Autodesk Fusion 360 part; units mm, degrees
(part 2 of 2)
extrude "Extrude179" add sketch "Sketch179" along normal blind 62 from surface at 3 bodies 3
sketch "Sketch180" plane through (0, 0, 0) normal (0, 0, 1) x (1, 0, 0)
  line L0 (-121.5, 16) -> (-128.5, 16)
  line L1 (-128.5, 16) -> (-128.5, 3)
  line L2 (-128.5, 3) -> (-121.5, 3)
  line L3 (-121.5, 3) -> (-121.5, 16)
extrude "Extrude180" add sketch "Sketch180" along normal blind 8 from surface at 57 bodies 3
sketch "Sketch181" plane through (0, 0, 0) normal (0, 0, 1) x (1, 0, 0)
  circle A0 centre (-125, 12) radius 1.3
extrude "Extrude181" cut sketch "Sketch181" along normal blind 8 from surface at 57 bodies 3
sketch "Sketch182" plane through (0, 0, 0) normal (0, 0, 1) x (1, 0, 0)
  line L0 (128.5, 16) -> (121.5, 16)
  line L1 (121.5, 16) -> (121.5, 3)
  line L2 (121.5, 3) -> (128.5, 3)
  line L3 (128.5, 3) -> (128.5, 16)
extrude "Extrude182" add sketch "Sketch182" along normal blind 8 from surface at 57 bodies 3
sketch "Sketch183" plane through (0, 0, 0) normal (0, 0, 1) x (1, 0, 0)
  circle A0 centre (125, 12) radius 1.3
extrude "Extrude183" cut sketch "Sketch183" along normal blind 8 from surface at 57 bodies 3
sketch "Sketch184" plane through (0, 0, 0) normal (0, 0, 1) x (1, 0, 0)
  line L0 (140, 83) -> (-140, 83)
  line L1 (-140, 83) -> (-140, 80)
  line L2 (-140, 80) -> (140, 80)
  line L3 (140, 80) -> (140, 83)
extrude "Extrude184" add sketch "Sketch184" along normal blind 3 bodies 3
sketch "Sketch185" plane through (0, 0, 0) normal (0, 0, 1) x (1, 0, 0)
  line L0 (125, 82.3) -> (-125, 82.3)
  line L1 (-125, 82.3) -> (-125, 80.7)
  line L2 (-125, 80.7) -> (125, 80.7)
  line L3 (125, 80.7) -> (125, 82.3)
extrude "Extrude185" cut sketch "Sketch185" along normal blind 2 from surface at 2 bodies 3
move_body "Move2" bodies 3 to x (-1, 0, 0) y (0, 0, 1) z (0, 1, 0) at (0, 137, 0)
sketch "Sketch186" plane through (0, 0, 0) normal (0, 0, 1) x (1, 0, 0)
  line L0 (140, 40) -> (-140, 40)
  line L1 (-140, 40) -> (-140, -40)
  line L2 (-140, -40) -> (140, -40)
  line L3 (140, -40) -> (140, 40)
extrude "Extrude186" add sketch "Sketch186" along normal blind 2.5 separate body makes body 4
sketch "Sketch187" plane through (0, 0, 0) normal (0, 0, 1) x (1, 0, 0)
  line L0 (94, -33) -> (87, -33)
  line L1 (87, -33) -> (87, -42)
  line L2 (87, -42) -> (94, -42)
  line L3 (94, -42) -> (94, -33)
extrude "Extrude187" cut sketch "Sketch187" along normal blind 2.95 from surface at -1 bodies 4
sketch "Sketch188" plane through (0, 0, 0) normal (0, 0, 1) x (1, 0, 0)
  circle A0 centre (90.5, -33) radius 3.5
extrude "Extrude188" cut sketch "Sketch188" along normal blind 2.95 from surface at -1 bodies 4
sketch "Sketch189" plane through (0, 0, 0) normal (0, 0, 1) x (1, 0, 0)
  line L0 (80, -33) -> (73, -33)
  line L1 (73, -33) -> (73, -42)
  line L2 (73, -42) -> (80, -42)
  line L3 (80, -42) -> (80, -33)
extrude "Extrude189" cut sketch "Sketch189" along normal blind 2.95 from surface at -1 bodies 4
sketch "Sketch190" plane through (0, 0, 0) normal (0, 0, 1) x (1, 0, 0)
  circle A0 centre (76.5, -33) radius 3.5
extrude "Extrude190" cut sketch "Sketch190" along normal blind 2.95 from surface at -1 bodies 4
sketch "Sketch191" plane through (0, 0, 0) normal (0, 0, 1) x (1, 0, 0)
  line L0 (66, -33) -> (59, -33)
  line L1 (59, -33) -> (59, -42)
  line L2 (59, -42) -> (66, -42)
  line L3 (66, -42) -> (66, -33)
extrude "Extrude191" cut sketch "Sketch191" along normal blind 2.95 from surface at -1 bodies 4
sketch "Sketch192" plane through (0, 0, 0) normal (0, 0, 1) x (1, 0, 0)
  circle A0 centre (62.5, -33) radius 3.5
extrude "Extrude192" cut sketch "Sketch192" along normal blind 2.95 from surface at -1 bodies 4
sketch "Sketch193" plane through (0, 0, 0) normal (0, 0, 1) x (1, 0, 0)
  line L0 (52, -33) -> (45, -33)
  line L1 (45, -33) -> (45, -42)
  line L2 (45, -42) -> (52, -42)
  line L3 (52, -42) -> (52, -33)
extrude "Extrude193" cut sketch "Sketch193" along normal blind 2.95 from surface at -1 bodies 4
sketch "Sketch194" plane through (0, 0, 0) normal (0, 0, 1) x (1, 0, 0)
  circle A0 centre (48.5, -33) radius 3.5
extrude "Extrude194" cut sketch "Sketch194" along normal blind 2.95 from surface at -1 bodies 4
sketch "Sketch195" plane through (0, 0, 0) normal (0, 0, 1) x (1, 0, 0)
  line L0 (38, -33) -> (31, -33)
  line L1 (31, -33) -> (31, -42)
  line L2 (31, -42) -> (38, -42)
  line L3 (38, -42) -> (38, -33)
extrude "Extrude195" cut sketch "Sketch195" along normal blind 2.95 from surface at -1 bodies 4
sketch "Sketch196" plane through (0, 0, 0) normal (0, 0, 1) x (1, 0, 0)
  circle A0 centre (34.5, -33) radius 3.5
extrude "Extrude196" cut sketch "Sketch196" along normal blind 2.95 from surface at -1 bodies 4
sketch "Sketch197" plane through (0, 0, 0) normal (0, 0, 1) x (1, 0, 0)
  line L0 (-99.5, -33) -> (-106.5, -33)
  line L1 (-106.5, -33) -> (-106.5, -42)
  line L2 (-106.5, -42) -> (-99.5, -42)
  line L3 (-99.5, -42) -> (-99.5, -33)
extrude "Extrude197" cut sketch "Sketch197" along normal blind 2.95 from surface at -1 bodies 4
sketch "Sketch198" plane through (0, 0, 0) normal (0, 0, 1) x (1, 0, 0)
  circle A0 centre (-103, -33) radius 3.5
extrude "Extrude198" cut sketch "Sketch198" along normal blind 2.95 from surface at -1 bodies 4
sketch "Sketch199" plane through (0, 0, 0) normal (0, 0, 1) x (1, 0, 0)
  line L0 (-83.5, -33) -> (-90.5, -33)
  line L1 (-90.5, -33) -> (-90.5, -42)
  line L2 (-90.5, -42) -> (-83.5, -42)
  line L3 (-83.5, -42) -> (-83.5, -33)
extrude "Extrude199" cut sketch "Sketch199" along normal blind 2.95 from surface at -1 bodies 4
sketch "Sketch200" plane through (0, 0, 0) normal (0, 0, 1) x (1, 0, 0)
  circle A0 centre (-87, -33) radius 3.5
extrude "Extrude200" cut sketch "Sketch200" along normal blind 2.95 from surface at -1 bodies 4
sketch "Sketch201" plane through (0, 0, 0) normal (0, 0, 1) x (1, 0, 0)
  line L0 (-67.5, -33) -> (-74.5, -33)
  line L1 (-74.5, -33) -> (-74.5, -42)
  line L2 (-74.5, -42) -> (-67.5, -42)
  line L3 (-67.5, -42) -> (-67.5, -33)
extrude "Extrude201" cut sketch "Sketch201" along normal blind 2.95 from surface at -1 bodies 4
sketch "Sketch202" plane through (0, 0, 0) normal (0, 0, 1) x (1, 0, 0)
  circle A0 centre (-71, -33) radius 3.5
extrude "Extrude202" cut sketch "Sketch202" along normal blind 2.95 from surface at -1 bodies 4
sketch "Sketch203" plane through (0, 0, 0) normal (0, 0, 1) x (1, 0, 0)
  line L0 (-51.5, -33) -> (-58.5, -33)
  line L1 (-58.5, -33) -> (-58.5, -42)
  line L2 (-58.5, -42) -> (-51.5, -42)
  line L3 (-51.5, -42) -> (-51.5, -33)
extrude "Extrude203" cut sketch "Sketch203" along normal blind 2.95 from surface at -1 bodies 4
sketch "Sketch204" plane through (0, 0, 0) normal (0, 0, 1) x (1, 0, 0)
  circle A0 centre (-55, -33) radius 3.5
extrude "Extrude204" cut sketch "Sketch204" along normal blind 2.95 from surface at -1 bodies 4
sketch "Sketch205" plane through (0, 0, 0) normal (0, 0, 1) x (1, 0, 0)
  line L0 (-35.5, -33) -> (-42.5, -33)
  line L1 (-42.5, -33) -> (-42.5, -42)
  line L2 (-42.5, -42) -> (-35.5, -42)
  line L3 (-35.5, -42) -> (-35.5, -33)
extrude "Extrude205" cut sketch "Sketch205" along normal blind 2.95 from surface at -1 bodies 4
sketch "Sketch206" plane through (0, 0, 0) normal (0, 0, 1) x (1, 0, 0)
  circle A0 centre (-39, -33) radius 3.5
extrude "Extrude206" cut sketch "Sketch206" along normal blind 2.95 from surface at -1 bodies 4
sketch "Sketch207" plane through (0, 0, 0) normal (0, 0, 1) x (1, 0, 0)
  line L0 (-6.5, -33) -> (-13.5, -33)
  line L1 (-13.5, -33) -> (-13.5, -42)
  line L2 (-13.5, -42) -> (-6.5, -42)
  line L3 (-6.5, -42) -> (-6.5, -33)
extrude "Extrude207" cut sketch "Sketch207" along normal blind 2.95 from surface at -1 bodies 4
sketch "Sketch208" plane through (0, 0, 0) normal (0, 0, 1) x (1, 0, 0)
  circle A0 centre (-10, -33) radius 3.5
extrude "Extrude208" cut sketch "Sketch208" along normal blind 2.95 from surface at -1 bodies 4
sketch "Sketch209" plane through (0, 0, 0) normal (0, 0, 1) x (1, 0, 0)
  line L0 (140, 40) -> (-140, 40)
  line L1 (-140, 40) -> (-140, 37.5)
  line L2 (-140, 37.5) -> (140, 37.5)
  line L3 (140, 37.5) -> (140, 40)
extrude "Extrude209" add sketch "Sketch209" along normal blind 65 bodies 4
sketch "Sketch210" plane through (0, 0, 0) normal (0, 0, 1) x (1, 0, 0)
  line L0 (124.5, 39) -> (-124.5, 39)
  line L1 (-124.5, 39) -> (-124.5, 38)
  line L2 (-124.5, 38) -> (124.5, 38)
  line L3 (124.5, 38) -> (124.5, 39)
extrude "Extrude210" add sketch "Sketch210" along normal blind 0.7 from surface at 65 bodies 4
sketch "Sketch211" plane through (0, 0, 0) normal (0, 0, 1) x (1, 0, 0)
  line L0 (-137.5, 40) -> (-140, 40)
  line L1 (-140, 40) -> (-140, -40)
  line L2 (-140, -40) -> (-137.5, -40)
  line L3 (-137.5, -40) -> (-137.5, 40)
extrude "Extrude211" add sketch "Sketch211" along normal blind 65 bodies 4
sketch "Sketch212" plane through (0, 0, 0) normal (0, 0, 1) x (1, 0, 0)
  line L0 (140, 40) -> (137.5, 40)
  line L1 (137.5, 40) -> (137.5, -40)
  line L2 (137.5, -40) -> (140, -40)
  line L3 (140, -40) -> (140, 40)
extrude "Extrude212" add sketch "Sketch212" along normal blind 65 bodies 4
sketch "Sketch213" plane through (0, 0, 0) normal (0, 0, 1) x (1, 0, 0)
  line L0 (-129.1, -31.7) -> (-136.9, -31.7)
  line L1 (-136.9, -31.7) -> (-136.9, -34.7)
  line L2 (-136.9, -34.7) -> (-129.1, -34.7)
  line L3 (-129.1, -34.7) -> (-129.1, -31.7)
extrude "Extrude213" add sketch "Sketch213" along normal blind 60.5 from surface at 2.5 bodies 4
sketch "Sketch214" plane through (0, 0, 0) normal (0, 0, 1) x (1, 0, 0)
  line L0 (-135.3, -34.7) -> (-136.9, -34.7)
  line L1 (-136.9, -34.7) -> (-136.9, -40)
  line L2 (-136.9, -40) -> (-135.3, -40)
  line L3 (-135.3, -40) -> (-135.3, -34.7)
extrude "Extrude214" add sketch "Sketch214" along normal blind 60.5 from surface at 2.5 bodies 4
sketch "Sketch215" plane through (0, 0, 0) normal (0, 0, 1) x (1, 0, 0)
  line L0 (-129.1, -34.7) -> (-130.7, -34.7)
  line L1 (-130.7, -34.7) -> (-130.7, -40)
  line L2 (-130.7, -40) -> (-129.1, -40)
  line L3 (-129.1, -40) -> (-129.1, -34.7)
extrude "Extrude215" add sketch "Sketch215" along normal blind 60.5 from surface at 2.5 bodies 4
sketch "Sketch216" plane through (0, 0, 0) normal (0, 0, 1) x (1, 0, 0)
  line L0 (136.9, -31.7) -> (129.1, -31.7)
  line L1 (129.1, -31.7) -> (129.1, -34.7)
  line L2 (129.1, -34.7) -> (136.9, -34.7)
  line L3 (136.9, -34.7) -> (136.9, -31.7)
extrude "Extrude216" add sketch "Sketch216" along normal blind 60.5 from surface at 2.5 bodies 4
sketch "Sketch217" plane through (0, 0, 0) normal (0, 0, 1) x (1, 0, 0)
  line L0 (130.7, -34.7) -> (129.1, -34.7)
  line L1 (129.1, -34.7) -> (129.1, -40)
  line L2 (129.1, -40) -> (130.7, -40)
  line L3 (130.7, -40) -> (130.7, -34.7)
extrude "Extrude217" add sketch "Sketch217" along normal blind 60.5 from surface at 2.5 bodies 4
sketch "Sketch218" plane through (0, 0, 0) normal (0, 0, 1) x (1, 0, 0)
  line L0 (136.9, -34.7) -> (135.3, -34.7)
  line L1 (135.3, -34.7) -> (135.3, -40)
  line L2 (135.3, -40) -> (136.9, -40)
  line L3 (136.9, -40) -> (136.9, -34.7)
extrude "Extrude218" add sketch "Sketch218" along normal blind 60.5 from surface at 2.5 bodies 4
sketch "Sketch219" plane through (0, 0, 0) normal (0, 0, 1) x (1, 0, 0)
  circle A0 centre (-125, -31) radius 1.7
extrude "Extrude219" cut sketch "Sketch219" along normal blind 4.5 from surface at -1 bodies 4
sketch "Sketch220" plane through (0, 0, 0) normal (0, 0, 1) x (1, 0, 0)
  circle A0 centre (125, -31) radius 1.7
extrude "Extrude220" cut sketch "Sketch220" along normal blind 4.5 from surface at -1 bodies 4
move_body "Move3" bodies 4 to x (1, 0, 0) y (0, 0, 1) z (0, -1, 0) at (0, 205, 43)
named bodies: "CHECK: ALL-UP shell / actual FIR_Shell tub (see-through)", "CHECK: ALL-UP top cap / actual FIR_Shell (see-through)", "CHECK: ALL-UP bottom lid (actual FIR_BottomLid)", "CHECK: ALL-UP curved cover (actual FIR_CurvedLid)"
